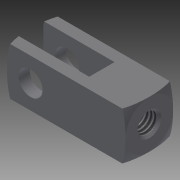
# Autodesk Inventor part: D-14043
Saved by Autodesk Inventor 2014 (Build 180170000, 170)
## iProperties
Created: 2014-01-19
Part Number: D-14043
Material: Generic
Catalog Web Link: www.cadenas.de
Description: Piston Rod Clevis for Original Line Cylinders - Body-
Vendor: BIMBA
Document SubType Name: Standard Catalog Part
Designer: Michael
Manufacturer: BIMBA
Density: 1 g/cm^3
Appearance: RGB(191.25000000000000,191.25000000000000,191.25000000000000)
Category: PARTsolutions
Company: BIMBA
Title: D-14043
Author: Cadenas PARTsolutions
PSOL_IDENT_0: {$CADENAS_DATA\23d-libs\bimba\bimba\bimba_imperial\bimba_full_line\original_line_cylinders\accessori
PSOL_IDENT_1: es\piston_rod_clevis_body.prj},203 {VTYP=3D},{NB=D-14043},{LINA=D-14043},{NN=Piston Rod Clevis for O
PSOL_IDENT_2: riginal Line Cylinders - Body},{DATE=06.12.2012 09:37:17},{GEOMDATE=06.12.2012 07:16:06},{VERSION=},
PSOL_IDENT_3: {LINEID=190},{LINESUBID=-1},{WBVAR=}  {NB=D-14043},{LINA=D-14043},{KT=DUMMY},{PN=D-14043},{L=0.93700
PSOL_IDENT_4: 000},{L1=0.75000000},{L2=0.37500000},{W=0.20000000},{W1=0.37500000},{DIA1=0.19000000},{DIA1CS=0.0000
PSOL_IDENT_5: 0000},{DIA2=0.37500000},{DIA3=0.15620000},{CS=90.00000000},{CDP=0.03000000},{AN=30.00000000},{NDM=0.
PSOL_IDENT_6: 19000000},{CODE=UNF},{NDMDP=0.31000000},{COLOR=0.75,0.75,0.75,0.00}
CNS_NN: Piston Rod Clevis for Original Line Cylinders - Body
CNS_NB: D-14043
CNS_NBSYN: $PN.
CNS_LINA: D-14043
CNS_PN: D-14043
CNS_L: 0.93700000
CNS_L1: 0.75000000
CNS_L2: 0.37500000
CNS_W: 0.20000000
CNS_W1: 0.37500000
CNS_DIA1: 0.19000000
CNS_DIA1CS: 0.00000000
CNS_DIA2: 0.37500000
CNS_DIA3: 0.15620000
CNS_CS: 90.00000000
CNS_CDP: 0.03000000
CNS_AN: 30.00000000
CNS_NDM: 0.19000000
CNS_CODE: UNF
CNS_NDMDP: 0.31000000
CNS_COLOR: 0.75,0.75,0.75,0.00
SUPPLIER: BIMBA
ARTICLENO: D-14043
BOMINFO: D-14043
CREATOR: CADENAS GmbH
Autodesk Inventor part; units mm, degrees
ref_plane "YZ Plane" through (0, 0, 0) normal (1, 0, 0) x (0, 1, 0)
ref_plane "XZ Plane" through (0, 0, 0) normal (0, 1, 0) x (-1, 0, 0)
ref_plane "XY Plane" through (0, 0, 0) normal (0, 0, 1) x (1, 0, 0)
sketch "Sketch_1" plane through (0, 0, 0) normal (0, 0, 1) x (1, 0, 0)
  line L0 (-4.7498, 4.7625) -> (-4.7498, -4.7625)
  line L1 (-4.7498, -4.7625) -> (19.05, -4.7625)
  line L2 (19.05, -4.7625) -> (19.05, 4.7625)
  line L3 (19.05, 4.7625) -> (-4.7498, 4.7625)
  constraints: 8 end point
extrude "Extrusion1" add sketch "Sketch_1" along normal mid plane 9.525
sketch "Sketch_2" plane through (0, 0, 0) normal (0, 1, 0) x (-1, 0, 0)
  line L0 (4.7498, -2.54) -> (4.7498, 2.54)
  line L1 (4.7498, 2.54) -> (-9.525, 2.54)
  line L2 (-9.525, 2.54) -> (-9.525, -2.54)
  line L3 (-9.525, -2.54) -> (4.7498, -2.54)
  constraints: 8 end point
extrude "Extrusion2" cut sketch "Sketch_2" along normal mid plane 9.525
sketch "Sketch3" plane through (19.05, -4.7625, 4.7625) normal (1, 0, 0) x (0, 0, -1)
  point P0 (4.7625, 4.7625)
hole "Hole1" at (19.05, 0, 0) direction (-1, 0, 0) diameter 3.9624 depth 7.874 countersink diameter 4.826 countersink angle 90 thread size "10-32 UNF" class "2B" standard "ANSI Unified Screw Threads"
sketch "Sketch4" plane through (11.176, 0, 0) normal (1, 0, 0) x (0, 0, -1)
  point P0 (0, 0)
hole "Hole2" at (11.176, 0, 0) direction (-1, 0, 0) diameter 3.9675 depth 1.651
sketch "Sketch5" plane through (0, 0, -4.7625) normal (0, 0, -1) x (-1, 0, 0)
  point P0 (0, 0)
hole "Hole3" at (0, 0, -4.7625) direction (0, 0, 1) diameter 4.826 depth 9.525
sketch "Sketch_9" plane through (0, 0, 0) normal (0, 0, 1) x (1, 0, 0)
  line L0 (23.8125, 0) -> (19.05, 0)
  line L1 (19.05, 0) -> (19.05, 4.7625)
  arc A0 (19.05, 4.7625) -> (16.51, 9.525) centre (8.8503, 2.3812) ccw
  line L2 (16.51, 9.525) -> (23.8125, 9.525)
  line L3 (23.8125, 9.525) -> (23.8125, 0)
  line L4 (23.8125, 0) -> (19.05, 0)
  constraints: 10 end point, 2 point on circle, 1 centre point
revolve "Revolution1" cut sketch "Sketch_9" angle 360 about axis through (23.8125, 0, 0) along (1, 0, 0)
sketch "Sketch_10" plane through (0, 0, 0) normal (0, 0, 1) x (1, 0, 0)
  line L0 (-4.7498, 0) -> (-9.5123, 0)
  line L1 (-9.5123, 0) -> (-9.5123, 9.525)
  line L2 (-9.5123, 9.525) -> (-2.2098, 9.525)
  arc A0 (-2.2098, 9.525) -> (-4.7498, 4.7625) centre (5.4499, 2.3812) ccw
  line L3 (-4.7498, 4.7625) -> (-4.7498, 0)
  line L4 (-4.7498, 0) -> (-9.5123, 0)
  constraints: 10 end point, 2 point on circle, 1 centre point
revolve "Revolution2" cut sketch "Sketch_10" angle 360 about axis through (-4.7498, 0, 0) along (1, 0, 0)
ref_plane "dummy_XY" through (0, 0, 0) normal (0, 0, 1) x (1, 0, 0)
ref_plane "dummy_YZ" through (0, 0, 0) normal (1, 0, 0) x (0, 1, 0)
ref_plane "dummy_ZX" through (0, 0, 0) normal (0, 1, 0) x (0, 0, 1)
ref_plane "h1_XY" through (-4.7498, 4.7625, 0) normal (0, 0, 1) x (1, 0, 0)
ref_plane "h1_YZ" through (-4.7498, 4.7625, 0) normal (1, 0, 0) x (0, 1, 0)
ref_plane "h1_ZX" through (-4.7498, 4.7625, 0) normal (0, 1, 0) x (0, 0, 1)
ref_plane "h2_XY" through (-4.7498, -4.7625, 0) normal (0, 0, 1) x (1, 0, 0)
ref_plane "h2_YZ" through (-4.7498, -4.7625, 0) normal (1, 0, 0) x (0, 1, 0)
ref_plane "h2_ZX" through (-4.7498, -4.7625, 0) normal (0, 1, 0) x (0, 0, 1)
ref_plane "l1_XY" through (19.05, 4.7625, 0) normal (0, 0, 1) x (1, 0, 0)
ref_plane "l1_YZ" through (19.05, 4.7625, 0) normal (1, 0, 0) x (0, 1, 0)
ref_plane "l1_ZX" through (19.05, 4.7625, 0) normal (0, 1, 0) x (0, 0, 1)
ref_plane "l11_XY" through (19.05, 4.7625, 0) normal (0, 0, 1) x (1, 0, 0)
ref_plane "l11_YZ" through (19.05, 4.7625, 0) normal (1, 0, 0) x (0, 1, 0)
ref_plane "l11_ZX" through (19.05, 4.7625, 0) normal (0, 1, 0) x (0, 0, 1)
ref_plane "l12_XY" through (0, 4.7625, 0) normal (0, 0, 1) x (1, 0, 0)
ref_plane "l12_YZ" through (0, 4.7625, 0) normal (1, 0, 0) x (0, 1, 0)
ref_plane "l12_ZX" through (0, 4.7625, 0) normal (0, 1, 0) x (0, 0, 1)
ref_plane "l2_XY" through (-4.7498, 4.7625, 0) normal (0, 0, 1) x (1, 0, 0)
ref_plane "l2_YZ" through (-4.7498, 4.7625, 0) normal (1, 0, 0) x (0, 1, 0)
ref_plane "l2_ZX" through (-4.7498, 4.7625, 0) normal (0, 1, 0) x (0, 0, 1)
ref_plane "l21_XY" through (19.05, 0, 0) normal (0, 1, 0) x (1, 0, 0)
ref_plane "l21_YZ" through (19.05, 0, 0) normal (1, 0, 0) x (0, 0, -1)
ref_plane "l21_ZX" through (19.05, 0, 0) normal (0, 0, -1) x (0, 1, 0)
ref_plane "l22_XY" through (9.525, 0, 0) normal (0, 1, 0) x (1, 0, 0)
ref_plane "l22_YZ" through (9.525, 0, 0) normal (1, 0, 0) x (0, 0, -1)
ref_plane "l22_ZX" through (9.525, 0, 0) normal (0, 0, -1) x (0, 1, 0)
ref_plane "piston_rod_clevis_XY" through (19.05, 0, 0) normal (1, 0, 0) x (0, 0, -1)
ref_plane "piston_rod_clevis_YZ" through (19.05, 0, 0) normal (0, 0, -1) x (0, 1, 0)
ref_plane "piston_rod_clevis_ZX" through (19.05, 0, 0) normal (0, 1, 0) x (1, 0, 0)
ref_plane "rod_clevis_body_XY" through (0, 0, 0) normal (0, 0, 1) x (1, 0, 0)
ref_plane "rod_clevis_body_YZ" through (0, 0, 0) normal (1, 0, 0) x (0, 1, 0)
ref_plane "rod_clevis_body_ZX" through (0, 0, 0) normal (0, 1, 0) x (0, 0, 1)
ref_plane "th1_XY" through (19.05, 2.413, 0) normal (0, 0, 1) x (1, 0, 0)
ref_plane "th1_YZ" through (19.05, 2.413, 0) normal (1, 0, 0) x (0, 1, 0)
ref_plane "th1_ZX" through (19.05, 2.413, 0) normal (0, 1, 0) x (0, 0, 1)
ref_plane "th2_XY" through (19.05, -2.413, 0) normal (0, 0, 1) x (1, 0, 0)
ref_plane "th2_YZ" through (19.05, -2.413, 0) normal (1, 0, 0) x (0, 1, 0)
ref_plane "th2_ZX" through (19.05, -2.413, 0) normal (0, 1, 0) x (0, 0, 1)
ref_plane "to_cylinder_XY" through (9.525, 0, 0) normal (1, 0, 0) x (0, 0, -1)
ref_plane "to_cylinder_YZ" through (9.525, 0, 0) normal (0, 0, -1) x (0, 1, 0)
ref_plane "to_cylinder_ZX" through (9.525, 0, 0) normal (0, 1, 0) x (1, 0, 0)
ref_plane "w1_XY" through (19.05, 0, -4.7625) normal (0, 1, 0) x (1, 0, 0)
ref_plane "w1_YZ" through (19.05, 0, -4.7625) normal (1, 0, 0) x (0, 0, -1)
ref_plane "w1_ZX" through (19.05, 0, -4.7625) normal (0, 0, -1) x (0, 1, 0)
ref_plane "w11_XY" through (-4.7498, 0, -2.54) normal (0, 1, 0) x (1, 0, 0)
ref_plane "w11_YZ" through (-4.7498, 0, -2.54) normal (1, 0, 0) x (0, 0, -1)
ref_plane "w11_ZX" through (-4.7498, 0, -2.54) normal (0, 0, -1) x (0, 1, 0)
ref_plane "w12_XY" through (-4.7498, 0, 2.54) normal (0, 1, 0) x (1, 0, 0)
ref_plane "w12_YZ" through (-4.7498, 0, 2.54) normal (1, 0, 0) x (0, 0, -1)
ref_plane "w12_ZX" through (-4.7498, 0, 2.54) normal (0, 0, -1) x (0, 1, 0)
ref_plane "w2_XY" through (19.05, 0, 4.7625) normal (0, 1, 0) x (1, 0, 0)
ref_plane "w2_YZ" through (19.05, 0, 4.7625) normal (1, 0, 0) x (0, 0, -1)
ref_plane "w2_ZX" through (19.05, 0, 4.7625) normal (0, 0, -1) x (0, 1, 0)
body "Solid1"
